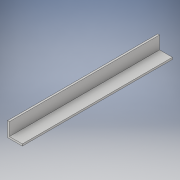
# Autodesk Inventor part: uchannel
Saved by Autodesk Inventor 2017 (Build 210142000, 142)
## iProperties
Created: 2018-10-17
Part Number: uchannel
Material: Generic
Document SubType Name: Modeling
Designer: ddeboer
Density: 1 g/cm^3
Appearance: Default
Author: ddeboer
Autodesk Inventor part; units mm, degrees
ref_plane "YZ Plane" through (0, 0, 0) normal (1, 0, 0) x (0, 1, 0)
ref_plane "XZ Plane" through (0, 0, 0) normal (0, 1, 0) x (-1, 0, 0)
ref_plane "XY Plane" through (0, 0, 0) normal (0, 0, 1) x (1, 0, 0)
sketch "Sketch1" plane through (0, 0, 0) normal (0, 0, 1) x (1, 0, 0)
  line L0 (0, 0) -> (25.4, 0)
  line L1 (0, 0) -> (0, 25.4)
  line L2 (3.175, 4.953) -> (3.175, 25.4)
  line L3 (3.175, 25.4) -> (0, 25.4)
  line L4 (4.953, 3.175) -> (25.4, 3.175)
  line L5 (25.4, 3.175) -> (25.4, 0)
  line L6 (3.175, 4.953) -> (3.175, 3.175)
  line L7 (3.175, 3.175) -> (4.953, 3.175)
  dimension "d6" = 25.4
  dimension "d7" = 25.4
  constraints: 16 end point, 3 perpendicular, 3 vertical, 2 horizontal
  measures "d6" distance of L0.start L0.end
  measures "d7" distance of L0.start L1.end
extrude "Extrusion1" add sketch "Sketch1" along normal blind 258.7752
body "Solid1"
